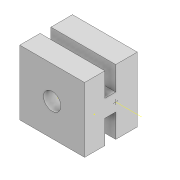
# Autodesk Inventor part: Corredera
Saved by Autodesk Inventor 2021 (Build 250183000, 183)
## iProperties
Created: 2021-07-04
Part Number: Corredera
Material: Generic
Document SubType Name: Modeling
Designer: Santiago
Density: 1 g/cm^3
Appearance: Default
Mass: 14.4487 g
Surface Area: 54.2566 cm^2
Volume: 14.4487 cm^3
Author: Santiago
Autodesk Inventor part; units mm, degrees
ref_plane "YZ Plane" through (0, 0, 0) normal (1, 0, 0) x (0, 1, 0)
ref_plane "XZ Plane" through (0, 0, 0) normal (0, 1, 0) x (-1, 0, 0)
ref_plane "XY Plane" through (0, 0, 0) normal (0, 0, 1) x (1, 0, 0)
sketch "Sketch1" plane through (0, 0, 0) normal (0, 0, 1) x (1, 0, 0)
  line L0 (15, -15) -> (-15, -15)
  line L1 (-15, -15) -> (-15, 15)
  line L2 (-15, 15) -> (15, 15)
  line L3 (15, 15) -> (15, -15)
  line L4 (15, -15) -> (-15, 15) construction
  line L5 (-15, -15) -> (15, 15) construction
  point P0 (0, 0)
  dimension "d0" = 30
  dimension "d1" = 30
  constraints: 12 end point, 2 midpoint, 2 parallel, 1 horizontal, 1 perpendicular
  measures "d0" distance of L1.end L2.end
  measures "d1" distance of L0.end L1.end
extrude "Extrusion1" add sketch "Sketch1" against normal blind 20
sketch "Sketch2" plane through (-15, 15, 0) normal (0, 1, 0) x (1, 0, 0)
  line L0 (30, 0) -> (30, 20) projected
  line L1 (0, 5) -> (30, 5)
  line L2 (30, 5) -> (30, 10)
  line L3 (30, 10) -> (0, 10)
  line L4 (0, 10) -> (0, 5)
  line L5 (0, 5) -> (30, 10) construction
  line L6 (30, 5) -> (0, 10) construction
  line L7 (0, 20) -> (30, 20) projected
  point P0 (15, 0)
  point P1 (15, 7.5)
  dimension "d4" = 5
  dimension "d13" = 10
  constraints: 12 end point, 3 midpoint, 2 parallel, 1 horizontal, 1 perpendicular
  measures "d4" distance of L2.end L1.end
  measures "d13" distance between parallel lines of L3 L7
extrude "Extrusion2" cut sketch "Sketch2" against normal blind 11
sketch "Sketch3" plane through (-15, -15, 0) normal (0, -1, 0) x (1, 0, 0)
  line L0 (30, 0) -> (30, -20) projected
  line L1 (0, -5) -> (30, -5)
  line L2 (30, -5) -> (30, -10)
  line L3 (30, -10) -> (0, -10)
  line L4 (0, -10) -> (0, -5)
  line L5 (0, -5) -> (30, -10) construction
  line L6 (30, -5) -> (0, -10) construction
  line L7 (30, -20) -> (0, -20) projected
  point P0 (15, 0)
  point P1 (15, -7.5)
  dimension "d7" = 5
  dimension "d14" = 10
  constraints: 12 end point, 3 midpoint, 2 parallel, 1 horizontal, 1 perpendicular
  measures "d7" distance of L1.end L2.end
  measures "d14" distance between parallel lines of L7 L3
extrude "Extrusion3" cut sketch "Sketch3" against normal blind 11
sketch "Sketch4" plane through (0, 0, 0) normal (0, 0, 1) x (1, 0, 0)
  circle A0 centre (0, 0) radius 4
  dimension "d10" = 8
  constraints: 1 centre point, 1 coincident
  measures "d10" diameter of A0
extrude "Extrusion4" cut sketch "Sketch4" against normal blind 5
sketch "Sketch5" plane through (15, -15, 0) normal (1, 0, 0) x (0, 0, -1)
  point P0 (0, 15)
  point P1 (10, 15)
sketch "Sketch6" plane through (0, 0, 0) normal (0, 0, 1) x (1, 0, 0)
  line L0 (15, 15) -> (-15, 15) projected
  line L1 (-15, 15) -> (-15, -15) projected
  circle A0 centre (0, 0) radius 4 projected
  line L2 (15, 15) -> (-15, 15) projected
  line L3 (-15, 15) -> (-15, -15) projected
  line L4 (-15, -15) -> (15, -15) projected
  line L5 (15, -15) -> (15, 15) projected
extrude "Extrusion5" add sketch "Sketch6" along normal blind 4.399
body "Solid1"
